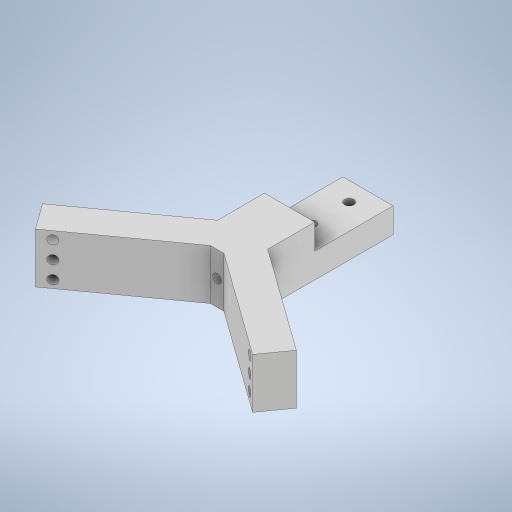
# Autodesk Inventor part: B1_head_T
Saved by Autodesk Inventor 2023.1 (Build 271208000, 208)
## iProperties
Created: 2023-06-14
Part Number: B1_head_T
Material: Generic
Document SubType Name: Modeling
Designer: zavrel
Density: 1 g/cm^3
Appearance: Default
Author: zavrel
Autodesk Inventor part; units mm, degrees
ref_plane "YZ Plane" through (0, 0, 0) normal (1, 0, 0) x (0, 1, 0)
ref_plane "XZ Plane" through (0, 0, 0) normal (0, 1, 0) x (-1, 0, 0)
ref_plane "XY Plane" through (0, 0, 0) normal (0, 0, 1) x (1, 0, 0)
sketch "Sketch1" plane through (0, 0, 0) normal (0, 1, 0) x (-1, 0, 0)
  line L0 (0, -50) -> (8, -50)
  line L1 (8, -50) -> (8, -10)
  line L2 (0, 0) -> (0, -50) construction
  line L3 (0, -50) -> (-8, -50)
  line L4 (-8, -50) -> (-8, -10)
  line L5 (8, -10) -> (40.4833, 13.3417)
  line L6 (40.4833, 13.3417) -> (34.6478, 21.4626)
  line L7 (34.6478, 21.4626) -> (2.1646, -1.8792)
  line L8 (2.1646, -1.8792) -> (0, -1.8792)
  line L9 (-8, -10) -> (-40.4833, 13.3417)
  line L10 (-40.4833, 13.3417) -> (-34.6478, 21.4626)
  line L11 (-34.6478, 21.4626) -> (-2.1646, -1.8792)
  line L12 (-2.1646, -1.8792) -> (0, -1.8792)
  point P0 (4, -50)
  dimension "d0" = 16
  dimension "d17" = 10
  dimension "d18" = 40
  constraints: 26 end point, 5 symmetric about line, 4 perpendicular, 1 horizontal, 1 midpoint, 1 point on line, 1 vertical
  measures "d0" distance between parallel lines of L4 L1
  measures "d17" distance between parallel lines of L7 L5
  measures "d18" distance of L1.end L5.end
extrude "Extrusion1" add sketch "Sketch1" along normal blind 16
sketch "Sketch2" plane through (0, 16, 0) normal (0, 1, 0) x (1, 0, 0)
  line L0 (8, 50) -> (-8, 50) projected
  line L1 (-8, 50) -> (-8, 10) projected
  line L2 (8, 10) -> (8, 50) projected
  line L3 (8, 10) -> (8, 50) projected
  line L4 (-8, 50) -> (8, 50)
  line L5 (8, 50) -> (8, 25)
  line L6 (8, 25) -> (-8, 25)
  line L7 (-8, 25) -> (-8, 50)
  line L8 (-8, 10) -> (-40.4833, -13.3417) projected
  line L9 (-40.4833, -13.3417) -> (-34.6478, -21.4626) projected
  line L10 (-34.6478, -21.4626) -> (-2.1646, 1.8792) projected
  line L11 (-2.1646, 1.8792) -> (2.1646, 1.8792) projected
  line L12 (2.1646, 1.8792) -> (34.6478, -21.4626) projected
  line L13 (34.6478, -21.4626) -> (40.4833, -13.3417) projected
  line L14 (40.4833, -13.3417) -> (8, 10) projected
  point P0 (0, 0)
  dimension "d6" = 25
  constraints: 8 end point, 2 parallel, 1 horizontal, 1 perpendicular, 1 point on line
  measures "d6" distance between parallel lines of L0 L6
extrude "Extrusion2" cut sketch "Sketch2" against normal blind 8 contours L2 L6 L1 L0
sketch "Sketch3" plane through (0, 0, 0) normal (0, -1, 0) x (1, 0, 0)
  line L0 (8, -50) -> (-8, -50) projected
  line L1 (8, -10) -> (8, -50) projected
  line L2 (-8, -50) -> (-8, -10) projected
  circle A0 centre (0, -44) radius 1.5
  circle A1 centre (0, -32) radius 1.5
  line L3 (40.4833, 13.3417) -> (8, -10) projected
  line L4 (34.6478, 21.4626) -> (40.4833, 13.3417) projected
  line L5 (2.1646, -1.8792) -> (34.6478, 21.4626) projected
  line L6 (-2.1646, -1.8792) -> (2.1646, -1.8792) projected
  line L7 (-34.6478, 21.4626) -> (-2.1646, -1.8792) projected
  line L8 (-40.4833, 13.3417) -> (-34.6478, 21.4626) projected
  line L9 (-8, -10) -> (-40.4833, 13.3417) projected
  point P0 (0, 0)
  dimension "d9" = 3
  dimension "d10" = 6
  dimension "d11" = 12
  constraints: 2 centre point, 1 equal radius
  measures "d9" diameter of A0
  measures "d10" distance from line of A0.centre L0
  measures "d11" distance of A0.centre A1.centre
extrude "Extrusion3" cut sketch "Sketch3" against normal through all contours A0 | A1
sketch "Sketch4" plane through (0, 0, 0) normal (0, -1, 0) x (1, 0, 0)
  circle A0 centre (0, -32) radius 1.5 projected
  circle A1 centre (0, -44) radius 1.5 projected
  line L0 (8, -50) -> (-8, -50) projected
  line L1 (8, -10) -> (8, -50) projected
  line L2 (-8, -50) -> (-8, -10) projected
  circle A2 centre (0, -44) radius 3
  circle A3 centre (0, -32) radius 1.5 projected
  circle A4 centre (0, -32) radius 3
  line L3 (40.4833, 13.3417) -> (8, -10) projected
  line L4 (34.6478, 21.4626) -> (40.4833, 13.3417) projected
  line L5 (2.1646, -1.8792) -> (34.6478, 21.4626) projected
  line L6 (-2.1646, -1.8792) -> (2.1646, -1.8792) projected
  line L7 (-34.6478, 21.4626) -> (-2.1646, -1.8792) projected
  line L8 (-40.4833, 13.3417) -> (-34.6478, 21.4626) projected
  line L9 (-8, -10) -> (-40.4833, 13.3417) projected
  point P0 (0, 0)
  dimension "d14" = 6
  constraints: 2 centre point, 2 coincident, 1 equal radius
  measures "d14" diameter of A4
extrude "Extrusion4" cut sketch "Sketch4" against normal blind 3 contours A2 | A4
sketch "Sketch5" plane through (-2.1646, 0, -1.8792) normal (0.5835436, 0, 0.8120818) x (0.8120818, 0, -0.5835436)
  line L0 (-40, 0) -> (0, 0) projected
  line L1 (0, 0) -> (0, 16) projected
  line L2 (-40, 16) -> (0, 16) projected
  line L3 (-40, 0) -> (-40, 16) projected
  line L4 (-40, 0) -> (-40, 16) construction
  line L5 (-40, 8) -> (0, 8) construction
  line L6 (0, 0) -> (0, 16) construction
  circle A0 centre (-36, 13.5) radius 1.4
  circle A1 centre (-36, 8) radius 1.4
  circle A2 centre (-36, 2.5) radius 1.4
  point P0 (0.6612, 0)
  dimension "d19" = 2.8
  dimension "d20" = 11
  dimension "d21" = 4
  constraints: 3 centre point, 2 end point, 2 midpoint, 1 equal radius, 1 point on line, 1 symmetric about line, 1 vertical alignment, 1 other
  measures "d19" diameter of A0
  measures "d20" distance of A2.centre A0.centre
  measures "d21" distance from line of L3 A1.centre
extrude "Extrusion5" cut sketch "Sketch5" against normal through all contours A0 | A1 | A2
sketch "Sketch7" plane through (-2.1646, 0, -1.8792) normal (0, 0, 1) x (1, 0, 0)
  line L0 (0, 0) -> (4.3291, 0) projected
  line L1 (4.3291, 0) -> (4.3291, 16) projected
  line L2 (0, 16) -> (4.3291, 16) projected
  line L3 (0, 0) -> (0, 16) projected
  line L4 (0, 0) -> (0, 16) construction
  line L5 (0, 8) -> (4.3291, 8) construction
  line L6 (0.6646, 8) -> (3.6646, 8) projected
  circle A0 centre (2.1646, 8) radius 1.4
  point P0 (2.1646, 0)
  dimension "d24" = 2.8
  constraints: 3 midpoint, 2 end point, 1 centre point
  measures "d24" diameter of A0
extrude "Extrusion6" cut sketch "Sketch7" against normal blind 20 contours A0 L6 | L6 A0
sketch "Sketch8" plane through (34.6478, 0, 21.4626) normal (-0.5835436, 0, 0.8120818) x (0.8120818, 0, 0.5835436)
  line L0 (-40, 0) -> (0, 0) projected
  line L1 (0, 0) -> (0, 16) projected
  line L2 (-40, 16) -> (0, 16) projected
  line L3 (-40, 0) -> (-40, 16) projected
  line L4 (0, 0) -> (0, 16) construction
  line L5 (0, 8) -> (-40, 8) construction
  line L6 (-40, 0) -> (-40, 16) construction
  circle A0 centre (-4, 8) radius 1.4
  circle A1 centre (-4, 3) radius 1.4
  circle A2 centre (-4, 13) radius 1.4
  point P0 (-40.6612, 0)
  dimension "d27" = 2.8
  dimension "d28" = 4
  dimension "d29" = 10
  constraints: 3 centre point, 2 end point, 2 midpoint, 2 vertical alignment, 1 equal radius, 1 point on line, 1 other
  measures "d27" diameter of A1
  measures "d28" distance from line of L1 A1.centre
  measures "d29" distance of A2.centre A1.centre
extrude "Extrusion7" cut sketch "Sketch8" against normal through all contours A0 | A1 | A2
body "Solid1"
